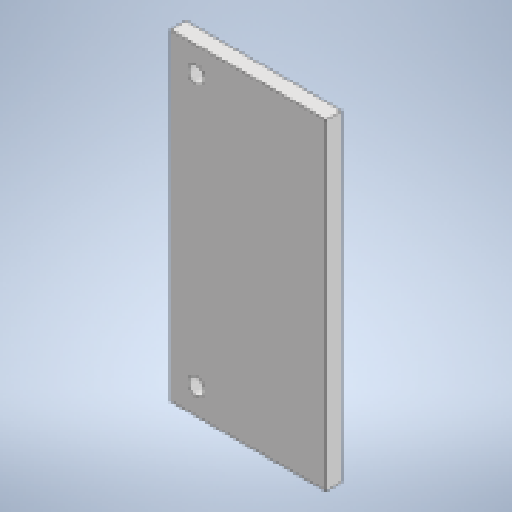
# Autodesk Inventor part: Lateral derecho
Saved by Autodesk Inventor 2024 (Build 280153000, 153)
## iProperties
Created: 2025-03-02
Part Number: Lateral derecho
Material: Genérico
Document SubType Name: Modeling
Designer: sergi
Density: 1 g/cm^3
Appearance: Valor por defecto
Author: sergi
Autodesk Inventor part; units mm, degrees
sketch "Boceto2" plane through (0, 0, 0) normal (1, 0, 0) x (0, 1, 0)
  line L0 (0, 0) -> (-67, 0)
  line L1 (-67, 0) -> (-67, 6)
  line L2 (-67, 6) -> (0, 6)
  line L3 (0, 6) -> (0, 0)
  dimension "d2" = 67
  dimension "d3" = 6
  constraints: 8 end point, 2 parallel, 1 horizontal, 1 perpendicular
  measures "d2" distance of L1.end L2.end
  measures "d3" distance of L0.end L1.end
extrude "Extrusión2" add sketch "Boceto2" along normal blind 65
sketch "Boceto3" plane through (65, 0, 0) normal (1, 0, 0) x (0, 0, -1)
  line L0 (-6, -5) -> (72, -5) projected
  line L1 (-6, -8) -> (-6, -5) projected
  line L2 (72, -8) -> (-6, -8) projected
  line L3 (72, -5) -> (72, -8) projected
  line L4 (-6, 0) -> (-6, -67) projected
  line L5 (-6, -67) -> (0, -67) projected
  line L6 (0, -67) -> (0, 0) projected
  line L7 (0, 0) -> (-6, 0) projected
  point P0 (0, -5)
ref_plane "Plano de trabajo1" through (31.12, -8, -69) normal (-1, 0, 0) x (0, 0, 1)
ref_plane "Plano de trabajo2" through (33.12, -8, -69) normal (-1, 0, 0) x (0, 0, 1)
ref_plane "Plano de trabajo4" through (31.12, -8, -72) normal (-1, 0, 0) x (0, 0, 1)
extrude "Extrusión3" cut sketch "Boceto3" against normal up to surface (33.88 mm away) contours L0 L6 L2 L1 | L2 L6 L5 L4
sketch "Boceto4" plane through (0, 0, 6) normal (0, 1, 0) x (1, 0, 0)
  circle A0 centre (34.12, 75) radius 1.5 projected
  circle A1 centre (62, 75) radius 1.5 projected
  line L0 (65, 0) -> (65, 78) projected
  line L1 (65, 78) -> (31.12, 78) projected
  line L2 (65, 0) -> (31.12, 0) projected
  line L3 (0, 6) -> (0, 0) projected
  line L4 (0, 0) -> (65, 0) projected
  line L5 (65, 6) -> (65, 0) projected
  line L6 (0, 6) -> (65, 6) projected
  line L7 (0, 0) -> (65, 0) projected
  line L8 (65, 0) -> (62, 0)
  line L9 (65, 0) -> (68, 0) construction
  line L10 (62, 0) -> (62, 3)
  circle A2 centre (62, 3) radius 2.1
  circle A3 centre (36.12, 3) radius 2.1
  circle A4 centre (36.12, 3) radius 1.5 projected
  circle A5 centre (62, 3) radius 1.5 projected
  line L11 (31.12, 0) -> (31.12, 78) projected
  point P0 (33.12, 0)
  dimension "d8" = 3
  dimension "d9" = 180
  dimension "d10" = 3
  dimension "d11" = 4.2
  dimension "d12" = 4.2
  constraints: 6 end point, 2 centre point, 2 horizontal, 1 coincident, 1 collinear, 1 perpendicular
  measures "d8" distance of L0.start L8.end
  measures "d9" angle of L9 L8
  measures "d10" distance of L8.end L10.end
  measures "d11" diameter of A2
  measures "d12" diameter of A3
hole "Agujero1" at (36.12, 0, 3) at (62, 0, 3) direction (0, -1, 0) diameter 4.2 depth 5
sketch "Boceto5" plane through (0, -67, 6) normal (0, 0, 1) x (1, 0, 0)
  circle A0 centre (5, 57) radius 2.1 projected
  circle A1 centre (5, 5) radius 2.1 projected
  point P0 (0, 67)
hole "Agujero2" at (5, -10, 6) at (5, -62, 6) direction (0, 0, -1) diameter 3.2 depth 5
sketch "Boceto6" plane through (31.12, -67, 6) normal (1, 0, 0) x (0, 0, -1)
  line L0 (6, 62) -> (0, 62) projected
  line L1 (0, 0) -> (0, 62) projected
  line L2 (6, 0) -> (0, 0) projected
  line L3 (6, 62) -> (6, 0) projected
  line L4 (6, 0) -> (3, 0)
  line L5 (3, 0) -> (3, 62)
  line L6 (3, 62) -> (6, 62)
  line L7 (6, 62) -> (6, 0)
  point P0 (6, 67)
  point P1 (3, 0)
  constraints: 8 end point, 2 parallel, 1 horizontal, 1 midpoint, 1 perpendicular
ref_plane "Plano de trabajo3" through (10, -67, -66) normal (1, 0, 0) x (0, 1, 0)
extrude "Extrusión4" cut sketch "Boceto6" against normal up to surface (21.12 mm away) contours L3 L2 L5 L0
sketch "Boceto7" plane through (31.12, -67, 6) normal (1, 0, 0) x (0, 0, -1)
  line L0 (3, 0) -> (3, 62) projected
  line L1 (3, 62) -> (0, 62) projected
  line L2 (0, 0) -> (0, 62) projected
  line L3 (3, 0) -> (0, 0) projected
  line L4 (0, 62) -> (78, 62) projected
  line L5 (0, 59) -> (0, 62) projected
  line L6 (78, 59) -> (0, 59) projected
  line L7 (78, 62) -> (78, 59) projected
  point P0 (6, 67)
  point P1 (3, 59)
extrude "Extrusión5" add sketch "Boceto7" along normal blind 6 contours L3 L2 L6 L0
